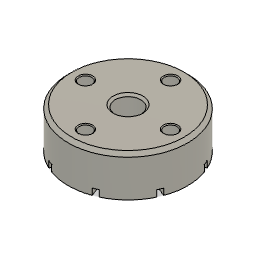
COLLAR (Autodesk Fusion 360 design; units mm, degrees)
Autodesk Fusion 360 part; units mm, degrees
sketch "Sketch1" plane through (0, 0, 0) normal (0, 1, 0) x (1, 0, 0)
  arc A0 (2.5733, 3.7888) -> (3.7888, 2.5733) centre (4.4176, 4.4176) ccw
  circle A1 centre (0, 0) radius 22.5
  arc A2 (2.6013, 4.6635) -> (2.5733, 3.7888) centre (3.747, 4.1889) ccw
  arc A3 (4.4987, -0.8595) -> (5.137, -1.4581) centre (5.6115, -0.3125) ccw
  arc A4 (-0.8595, 4.4987) -> (0.8595, 4.4987) centre (0, 6.2474) ccw
  arc A5 (0.8595, 4.4987) -> (1.4581, 5.137) centre (0.3125, 5.6115) ccw
  arc A6 (-1.4581, 5.137) -> (-0.8595, 4.4987) centre (-0.3125, 5.6115) ccw
  arc A7 (5.137, 1.4581) -> (4.4987, 0.8595) centre (5.6115, 0.3125) ccw
  arc A8 (-5.3666, -19.6149) -> (5.3666, -19.6149) centre (0, -7.8506) ccw
  line L0 (-5.137, -1.4581) -> (-17.0299, -6.3843)
  arc A9 (5.3666, 19.6149) -> (-5.3666, 19.6149) centre (0, 7.8506) ccw
  arc A10 (4.4987, 0.8595) -> (4.4987, -0.8595) centre (6.2474, 0) ccw
  line L1 (5.137, 1.4581) -> (17.0299, 6.3843)
  line L2 (-16.5563, -7.5275) -> (-4.6635, -2.6013)
  line L3 (-7.5275, 16.5563) -> (-2.6013, 4.6635)
  line L4 (-1.4581, 5.137) -> (-6.3843, 17.0299)
  arc A11 (-7.5275, 16.5563) -> (-10.075, 17.6646) centre (-9.3753, 15.791) ccw
  line L5 (17.0299, -6.3843) -> (5.137, -1.4581)
  line L6 (16.5563, 7.5275) -> (4.6635, 2.6013)
  arc A12 (-10.075, -17.6646) -> (-7.5275, -16.5563) centre (-9.3753, -15.791) ccw
  line L7 (-6.3843, -17.0299) -> (-1.4581, -5.137)
  arc A13 (-2.5733, 3.7888) -> (-2.6013, 4.6635) centre (-3.747, 4.1889) ccw
  arc A14 (-5.3666, 19.6149) -> (-6.3843, 17.0299) centre (-4.5366, 17.7952) ccw
  arc A15 (-17.6646, 10.075) -> (-16.5563, 7.5275) centre (-15.791, 9.3753) ccw
  arc A16 (-3.7888, 2.5733) -> (-2.5733, 3.7888) centre (-4.4176, 4.4176) ccw
  line L8 (-17.0299, 6.3843) -> (-5.137, 1.4581)
  arc A17 (-10.075, 17.6646) -> (-17.6646, 10.075) centre (-5.5512, 5.5512) ccw
  arc A18 (0.8595, -4.4987) -> (-0.8595, -4.4987) centre (0, -6.2474) ccw
  arc A19 (6.3843, 17.0299) -> (5.3666, 19.6149) centre (4.5366, 17.7952) ccw
  line L9 (-2.6013, -4.6635) -> (-7.5275, -16.5563)
  arc A20 (-16.5563, -7.5275) -> (-17.6646, -10.075) centre (-15.791, -9.3753) ccw
  line L10 (1.4581, -5.137) -> (6.3843, -17.0299)
  arc A21 (1.4581, -5.137) -> (0.8595, -4.4987) centre (0.3125, -5.6115) ccw
  line L11 (2.6013, 4.6635) -> (7.5275, 16.5563)
  line L12 (6.3843, 17.0299) -> (1.4581, 5.137)
  arc A22 (-6.3843, -17.0299) -> (-5.3666, -19.6149) centre (-4.5366, -17.7952) ccw
  arc A23 (-0.8595, -4.4987) -> (-1.4581, -5.137) centre (-0.3125, -5.6115) ccw
  arc A24 (-3.7888, -2.5733) -> (-4.6635, -2.6013) centre (-4.1889, -3.747) ccw
  arc A25 (-2.6013, -4.6635) -> (-2.5733, -3.7888) centre (-3.747, -4.1889) ccw
  arc A26 (-17.6646, -10.075) -> (-10.075, -17.6646) centre (-5.5512, -5.5512) ccw
  arc A27 (-2.5733, -3.7888) -> (-3.7888, -2.5733) centre (-4.4176, -4.4176) ccw
  line L13 (-4.6635, 2.6013) -> (-16.5563, 7.5275)
  arc A28 (17.6646, 10.075) -> (10.075, 17.6646) centre (5.5512, 5.5512) ccw
  arc A29 (-19.6149, -5.3666) -> (-17.0299, -6.3843) centre (-17.7952, -4.5366) ccw
  arc A30 (-17.0299, 6.3843) -> (-19.6149, 5.3666) centre (-17.7952, 4.5366) ccw
  arc A31 (-19.6149, 5.3666) -> (-19.6149, -5.3666) centre (-7.8506, 0) ccw
  arc A32 (5.3666, -19.6149) -> (6.3843, -17.0299) centre (4.5366, -17.7952) ccw
  arc A33 (16.5563, 7.5275) -> (17.6646, 10.075) centre (15.791, 9.3753) ccw
  arc A34 (-4.6635, 2.6013) -> (-3.7888, 2.5733) centre (-4.1889, 3.747) ccw
  arc A35 (-4.4987, -0.8595) -> (-4.4987, 0.8595) centre (-6.2474, 0) ccw
  arc A36 (-5.137, -1.4581) -> (-4.4987, -0.8595) centre (-5.6115, -0.3125) ccw
  arc A37 (-4.4987, 0.8595) -> (-5.137, 1.4581) centre (-5.6115, 0.3125) ccw
  arc A38 (10.075, 17.6646) -> (7.5275, 16.5563) centre (9.3753, 15.791) ccw
  arc A39 (19.6149, -5.3666) -> (19.6149, 5.3666) centre (7.8506, 0) ccw
  arc A40 (3.7888, -2.5733) -> (2.5733, -3.7888) centre (4.4176, -4.4176) ccw
  arc A41 (19.6149, 5.3666) -> (17.0299, 6.3843) centre (17.7952, 4.5366) ccw
  arc A42 (4.6635, -2.6013) -> (3.7888, -2.5733) centre (4.1889, -3.747) ccw
  line L14 (4.6635, -2.6013) -> (16.5563, -7.5275)
  arc A43 (17.6646, -10.075) -> (16.5563, -7.5275) centre (15.791, -9.3753) ccw
  line L15 (7.5275, -16.5563) -> (2.6013, -4.6635)
  arc A44 (2.5733, -3.7888) -> (2.6013, -4.6635) centre (3.747, -4.1889) ccw
  arc A45 (7.5275, -16.5563) -> (10.075, -17.6646) centre (9.3753, -15.791) ccw
  arc A46 (10.075, -17.6646) -> (17.6646, -10.075) centre (5.5512, -5.5512) ccw
  arc A47 (17.0299, -6.3843) -> (19.6149, -5.3666) centre (17.7952, -4.5366) ccw
  circle A48 centre (0, 0) radius 3
  circle A49 centre (0, 0) radius 3
  circle A50 centre (0, 0) radius 3.65
  arc A51 (3.7888, 2.5733) -> (4.6635, 2.6013) centre (4.1889, 3.747) ccw
  line L16 (-2.9593, 5.5277) -> (-5.2554, 11.071)
  line L17 (-2.9593, 5.5277) -> (-1.8161, 6.0012)
  line L18 (-1.8161, 6.0012) -> (-4.1122, 11.5445)
  line L19 (-5.2554, 11.071) -> (-4.1122, 11.5445)
  line L20 (-11.5445, 4.1122) -> (-11.071, 5.2554)
  line L21 (-6.0012, 1.8161) -> (-5.5277, 2.9593)
  line L22 (-11.071, -5.2554) -> (-11.5445, -4.1122)
  line L23 (-5.5277, -2.9593) -> (-6.0012, -1.8161)
  line L24 (-4.1122, -11.5445) -> (-5.2554, -11.071)
  line L25 (-1.8161, -6.0012) -> (-2.9593, -5.5277)
  line L26 (5.2554, -11.071) -> (4.1122, -11.5445)
  line L27 (2.9593, -5.5277) -> (1.8161, -6.0012)
  line L28 (11.5445, -4.1122) -> (11.071, -5.2554)
  line L29 (6.0012, -1.8161) -> (5.5277, -2.9593)
  line L30 (11.071, 5.2554) -> (11.5445, 4.1122)
  line L31 (5.5277, 2.9593) -> (6.0012, 1.8161)
  line L32 (4.1122, 11.5445) -> (5.2554, 11.071)
  line L33 (1.8161, 6.0012) -> (2.9593, 5.5277)
  circle A52 centre (0, 0) radius 14
  dimension "d1" = 6
  dimension "d2" = 7.3
  dimension "d3" = 6
  dimension "d4" = 6
  dimension "d6" = 360
  dimension "d7" = 28
  constraint coincident A1.centre A48.centre
  constraint coincident L3 L16.start
  constraint parallel L3 L16
  constraint coincident L4 L17.end
  constraint perpendicular L4 L17
  constraint perpendicular L17 L18
  constraint perpendicular L4 L19
  constraint concentric A50 A52
  measures "d1" diameter of A48
  measures "d2" diameter of A50
  measures "d3" distance of L16.start L16.end
  measures "d4" distance of L17.end L18.end
  measures "d7" diameter of A52
extrude "Extrude3" add sketch "Sketch1" along normal blind 1.5 contours A0 A2 L6 L11 A51 A52 | A4 A5 A6 L4 L12 L18 A52 | A3 A7 A10 L1 L5 A52 | L3 A13 A16 L13 A34 L16 A52 | A40 A42 L14 L15 A44 A52 | L0 L8 A35 A36 A37 A52 | L7 A18 L10 A21 A23 A52 | L2 L9 A24 A25 A27 A52 makes body 1 at (-8.08, 0, 0.325) makes body 2 at (8.08, 0, -0.325) makes body 3 at (5.4836, 0, -5.9432) makes body 4 at (-5.4836, 0, 5.9432) makes body 5 at (-5.9432, 0, -5.4836) makes body 6 at (5.9432, 0, 5.4836) makes body 7 at (-0.325, 1.5, -8.08) makes body 8 at (0.325, 0, 8.08)
sketch "Sketch3" plane through (0, 1.5, 0) normal (0, 1, 0) x (-1, 0, 0)
  arc A0 (-1.4581, 5.137) -> (-0.8595, 4.4987) centre (-0.3125, 5.6115) ccw
  arc A1 (-0.8595, 4.4987) -> (0.8595, 4.4987) centre (0, 6.2474) ccw
  arc A2 (0.8595, 4.4987) -> (1.4581, 5.137) centre (0.3125, 5.6115) ccw
  line L0 (1.4581, 5.137) -> (4.7807, 13.1584)
  arc A3 (4.7807, 13.1584) -> (-4.7807, 13.1584) centre (0, 0) ccw
  line L1 (-4.7807, 13.1584) -> (-1.4581, 5.137)
  circle A4 centre (0, 0) radius 3
  circle A5 centre (0, 0) radius 14
  dimension "d15" = 6
  constraint concentric A3 A4
  constraint concentric A4 A5
  measures "d15" diameter of A4
extrude "Extrude4" add sketch "Sketch3" along normal blind 8 contours A0 A1 A2 L0 A3 L1 A5 | A0 A1 A2 L0 L1 A5 | A4 bodies 1 2 3 4 5 6 7 8
chamfer "Chamfer1" distance 0.8 angle 45 1 edges at (13.0526, 9.5, -5.0626) on bodies 1
sketch "Sketch4" plane through (0, 9.5, 0) normal (0, 1, 0) x (-1, 0, 0)
  circle A0 centre (0, 0) radius 13.2
  circle A1 centre (0, 0) radius 3
  dimension "d19" = 6
  constraint coincident A0.centre A1.centre
  measures "d19" diameter of A1
extrude "Extrude5" cut sketch "Sketch4" against normal blind 41 contours A1 bodies 1
chamfer "Chamfer2" distance 0.5 angle 45 1 edges at (2.797, 9.5, 1.0848) on bodies 1
sketch "Sketch5" plane through (0, 9.5, 0) normal (0, 1, 0) x (-1, 0, 0)
  circle A0 centre (0, 0) radius 13.2
  circle A1 centre (0, 0) radius 3.5
  circle A2 centre (0, 10) radius 1.5
  circle A3 centre (-10, 0) radius 1.5
  circle A4 centre (0, -10) radius 1.5
  circle A5 centre (10, 0) radius 1.5
  dimension "d23" = 3
  dimension "d25" = 360
  measures "d23" diameter of A2
extrude "Extrude6" cut sketch "Sketch5" against normal blind 24 contours A2 | A3 | A4 | A5 bodies 1
chamfer "Chamfer3" distance 0.2 angle 45 4 edges at (-8.6015, 9.5, 0.5424) (1.3985, 9.5, -9.4576) (11.3985, 9.5, 0.5424) (1.3985, 9.5, 10.5424) on bodies 1
